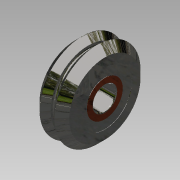
# Autodesk Inventor part: W3SSX
Saved by Autodesk Inventor 2020.1 (Build 241239000, 239)
## iProperties
Created: 2019-11-28
Part Number: W3SSX
Material: Generic
Catalog Web Link: https://www.bwc.com/dualvee.html
Description: Original DualVee Wheels-Original DualVee Wheels
Vendor: Bishop Wisecarver
Document SubType Name: Modeling
Designer: Autodesk Inc.
Manufacturer: BWC
Mass: 130.2 g
Surface Area: 59.8551 cm^2
Volume: 19.8505 cm^3
Density: 1 g/cm^3
Appearance: PSOLRGB-175-175-175
Category: FIRSTChoice
Company: Autodesk Inc.
PSOL_IDENT_0: {$CADENAS_DATA\23d-libs\bwc\dual_vee\wheels\original_dualvee_wheels.prj},168 {VTYP=3D},{NB=W3SSX},{L
PSOL_IDENT_1: INA=W3SSX},{NN=Original DualVee Wheels},{DATE=01.07.2019 05:07:11},{GEOMDATE=12.02.2019 13:07:27},{V
PSOL_IDENT_2: ERSION=},{LINEID=210},{WBVAR=},{WBNUMERIC=}  {NB=W3SSX},{LINA=W3SSX},{KT=DUMMY},{PN=W3SSX},{WS=WSSX
PSOL_IDENT_3: Stainless Steel Seal/Shield},{WSPN=SSX},{WSALG= 'X','WX Seal/Shield Steel', 'SSX','WSSX Seal/Shield
PSOL_IDENT_4: Stainless Steel','SS227', 'WSS227 Shield Stainless Steel Krytox GPL227 Lubricant','SS300', 'WSS300 S
PSOL_IDENT_5: tainless Steel Isoflex PDL 300 (grease, no shields or seals)','DW3SSX', 'Washdown Sealed Wheels' },{
PSOL_IDENT_6: SIZE=3},{D=1.803},{W=0.625},{B=0.4724},{VRI=0.750},{VRO=1.063},{WEIGHT=130.2},{C=0.755},{R=0.039},{R
PSOL_IDENT_7: 1=0.024},{E=0.010},{RLN=5900},{RLLBF=1326},{ALN=1701},{ALLBF=382},{ORMAT=440C Stainless steel},{IRMA
PSOL_IDENT_8: T=440C Stainless steel},{BMAT=440C Stainless steel},{RMAT=Nylon 6,6},{SHMAT=304 Stainless steel},{SM
PSOL_IDENT_9: AT=NBR+304 Stainless steel},{GREASE=Kluberplex BEM 34-132},{CFGFILTER=PN,WS,SIZE,D,W,B,VRI,VRO,WEIGH
PSOL_IDENT_10: T,RLN,RLLBF,ALN,ALLBF,ORMAT,IRMAT,BMAT,RMAT,SHMAT,SMAT,GREASE},{CATEGALG=Original Guide Wheel, Size
PSOL_IDENT_11: 3, Stainless Steel, Sealed/Shielded},{FEATALG=<li style=\" margin-top:0px; margin-bottom:0px; margin
PSOL_IDENT_12: -left:0px; margin-right:0px; -qt-block-indent:0; text-indent:0px;\"><span style=\" font-size:11pt; f
PSOL_IDENT_13: ont-weight:600;\">Corrosion resistant AISI 440C stainless steel</span></li><li style=\" font-size:11
PSOL_IDENT_14: pt; font-weight:600;\" style=\" margin-top:0px; margin-bottom:0px; margin-left:0px; margin-right:0px
PSOL_IDENT_15: ; -qt-block-indent:0; text-indent:0px;\">Double row angular contact ball bearing</li><li style=\" fo
PSOL_IDENT_16: nt-size:11pt; font-weight:600;\" style=\" margin-top:0px; margin-bottom:0px; margin-left:0px; margin
PSOL_IDENT_17: -right:0px; -qt-block-indent:0; text-indent:0px;\">Precision ground 90° vee inside or outside runnin
PSOL_IDENT_18: g surfaces</li><li style=\" font-size:11pt; font-weight:600;\" style=\" margin-top:0px; margin-botto
PSOL_IDENT_19: m:0px; margin-left:0px; margin-right:0px; -qt-block-indent:0; text-indent:0px;\">Hardened for heavy
PSOL_IDENT_20: loads and durability</li><li style=\" font-size:11pt; font-weight:600;\" style=\" margin-top:0px; ma
PSOL_IDENT_21: rgin-bottom:0px; margin-left:0px; margin-right:0px; -qt-block-indent:0; text-indent:0px;\">Seal/Shie
PSOL_IDENT_22: ld combination to protect against contamination</li>},{DESCRALG=<span style=\" font-size:11pt; font-
PSOL_IDENT_23: weight:600;\">DualVee WSSX series guide wheels are linear guide bearings with double row angular con
PSOL_IDENT_24: tact ball bearing arrangement.  Precision ground 90° vee inside or outside surfaces can be employed
PSOL_IDENT_25: to support loads and provide smooth and quiet motion. Use with DualVee guide track for linear motion
PSOL_IDENT_26: . Hybrid seal/shield design with rubber inner seal and metal outer shield protects against particle
PSOL_IDENT_27: contamination of all sizes. Through bore allows mounting on bushings or journals. Internally lubrica
PSOL_IDENT_28: ted with general purpose grease. </span>},{RATINGSALG=<span style=\" font-size:11pt; font-weight:600
PSOL_IDENT_29: ; color:#000000;\">Temperature Range:</span><span style=\" font-size:11pt; color:#000000;\"> -22°F t
PSOL_IDENT_30: o +212°F</span></p><p style=\" margin-top:0px; margin-bottom:0px; margin-left:0px; margin-right:0px;
PSOL_IDENT_31: -qt-block-indent:0; text-indent:0px;\"><span style=\" font-size:11pt; font-weight:600; color:#00000
PSOL_IDENT_32: 0;\">RoHS Compliant</span>},{MATCOLALG=ORMAT( title=\"$var. ($desc.)\", format=\"$value(SRC=VALDESC)
PSOL_IDENT_33: .\" ),IRMAT( title=\"$var. ($desc.)\", format=\"$value(SRC=VALDESC).\" ),BMAT( title=\"$var. ($desc.
PSOL_IDENT_34: )\", format=\"$value(SRC=VALDESC).\" ),RMAT( title=\"$var. ($desc.)\", format=\"$value(SRC=VALDESC).
PSOL_IDENT_35: \" ),SHMAT( title=\"$var. ($desc.)\", format=\"$value(SRC=VALDESC).\" ),SMAT( title=\"$var. ($desc.)
PSOL_IDENT_36: \", format=\"$value(SRC=VALDESC).\" ),GREASE( title=\"$var. ($desc.)\", format=\"$value(SRC=VALDESC)
PSOL_IDENT_37: .\" )},{MATCOL1=ORMAT( title=\"$var. ($desc.)\", format=\"$value(SRC=VALDESC).\" ),IRMAT( title=\"$v
PSOL_IDENT_38: ar. ($desc.)\", format=\"$value(SRC=VALDESC).\" ),BMAT( title=\"$var. ($desc.)\", format=\"$value(SR
PSOL_IDENT_39: C=VALDESC).\" ),RMAT( title=\"$var. ($desc.)\", format=\"$value(SRC=VALDESC).\" ),SHMAT( title=\"$va
PSOL_IDENT_40: r. ($desc.)\", format=\"$value(SRC=VALDESC).\" ),SMAT( title=\"$var. ($desc.)\", format=\"$value(SRC=
PSOL_IDENT_41: VALDESC).\" ),GREASE( title=\"$var. ($desc.)\", format=\"$value(SRC=VALDESC).\" )}
NN: Original DualVee Wheels
NT: Original DualVee Wheels
NB: W3SSX
NBSYN: $PN.
LINA: W3SSX
PN: W3SSX
WS: WSSX Stainless Steel Seal/Shield
SIZE: 3
D: 1.803
W: 0.625
B: 0.4724
VRI: 0.75
VRO: 1.063
WEIGHT: 130.2
RLN: 5900
RLLBF: 1326
ALN: 1701
ALLBF: 382
ORMAT: 440C Stainless steel
IRMAT: 440C Stainless steel
BMAT: 440C Stainless steel
RMAT: Nylon 6,6
SHMAT: 304 Stainless steel
SMAT: NBR+304 Stainless steel
GREASE: Kluberplex BEM 34-132
SUPPLIER: BWC
ARTICLENO: W3SSX
BOMINFO: W3SSX
CREATOR: CADENAS GmbH
Title: W3SSX
Author: Autodesk Inc.
Comments: Original DualVee Wheels
Autodesk Inventor part; units mm, degrees
sketch "Sketch_1" plane through (0, 0, 0) normal (0, 0, 1) x (1, 0, 0)
  line L0 (7.3279, 0) -> (-7.3279, 0)
  line L1 (-7.9375, 9.5885) -> (-7.9375, 6.6091)
  arc A0 (-7.9375, 6.6091) -> (-7.3279, 5.9995) centre (-7.3279, 6.6091) ccw
  line L2 (-7.3279, 5.9995) -> (7.3279, 5.9995)
  arc A1 (7.3279, 5.9995) -> (7.9375, 6.6091) centre (7.3279, 6.6091) ccw
  line L3 (7.9375, 6.6091) -> (7.9375, 9.5885)
  line L4 (7.9375, 9.5885) -> (7.8105, 9.5885)
  line L5 (7.8105, 9.5885) -> (7.8105, 9.4615)
  line L6 (7.8105, 9.4615) -> (7.6835, 9.4615)
  line L7 (7.6835, 9.4615) -> (7.6835, 14.4463)
  line L8 (7.6835, 14.4463) -> (7.8105, 14.4463)
  line L9 (7.8105, 14.4463) -> (7.8105, 14.3193)
  line L10 (7.8105, 14.3193) -> (7.9375, 14.3193)
  line L11 (7.9375, 14.3193) -> (7.9375, 19.05)
  line L12 (7.9375, 19.05) -> (4.0894, 22.8981)
  line L13 (4.0894, 22.8981) -> (3.8354, 22.8981)
  line L14 (3.8354, 22.8981) -> (0.9906, 20.0533)
  line L15 (0.9906, 20.0533) -> (0.9906, 19.05)
  arc A2 (-0.9906, 19.05) -> (0.9906, 19.05) centre (0, 19.05) ccw
  line L16 (-0.9906, 19.05) -> (-0.9906, 20.0533)
  line L17 (-0.9906, 20.0533) -> (-3.8354, 22.8981)
  line L18 (-3.8354, 22.8981) -> (-4.0894, 22.8981)
  line L19 (-4.0894, 22.8981) -> (-7.9375, 19.05)
  line L20 (-7.9375, 19.05) -> (-7.9375, 14.3193)
  line L21 (-7.9375, 14.3193) -> (-7.8105, 14.3193)
  line L22 (-7.8105, 14.3193) -> (-7.8105, 14.4463)
  line L23 (-7.8105, 14.4463) -> (-7.6835, 14.4463)
  line L24 (-7.6835, 14.4463) -> (-7.6835, 9.4615)
  line L25 (-7.6835, 9.4615) -> (-7.8105, 9.4615)
  line L26 (-7.8105, 9.4615) -> (-7.8105, 9.5885)
  line L27 (-7.8105, 9.5885) -> (-7.9375, 9.5885)
  constraints: 56 end point, 6 point on circle, 3 centre point
revolve "Revolution1" add sketch "Sketch_1" angle 360 about axis through (7.3279, 0, 0) along (1, 0, 0)
ref_plane "b_XY" through (-7.3279, 5.9995, 0) normal (0, 0, 1) x (1, 0, 0)
ref_plane "b_YZ" through (-7.3279, 5.9995, 0) normal (1, 0, 0) x (0, 1, 0)
ref_plane "b_ZX" through (-7.3279, 5.9995, 0) normal (0, 1, 0) x (0, 0, 1)
ref_plane "b1_XY" through (-7.3279, -5.9995, 0) normal (0, 0, 1) x (1, 0, 0)
ref_plane "b1_YZ" through (-7.3279, -5.9995, 0) normal (1, 0, 0) x (0, 1, 0)
ref_plane "b1_ZX" through (-7.3279, -5.9995, 0) normal (0, 1, 0) x (0, 0, 1)
ref_plane "d_XY" through (-3.9688, 22.8981, 0) normal (0, 0, 1) x (1, 0, 0)
ref_plane "d_YZ" through (-3.9688, 22.8981, 0) normal (1, 0, 0) x (0, 1, 0)
ref_plane "d_ZX" through (-3.9688, 22.8981, 0) normal (0, 1, 0) x (0, 0, 1)
ref_plane "d1_XY" through (-3.9688, -22.8981, 0) normal (0, 0, 1) x (1, 0, 0)
ref_plane "d1_YZ" through (-3.9688, -22.8981, 0) normal (1, 0, 0) x (0, 1, 0)
ref_plane "d1_ZX" through (-3.9688, -22.8981, 0) normal (0, 1, 0) x (0, 0, 1)
ref_plane "vri_XY" through (0, 19.05, 0) normal (0, 0, 1) x (1, 0, 0)
ref_plane "vri_YZ" through (0, 19.05, 0) normal (1, 0, 0) x (0, 1, 0)
ref_plane "vri_ZX" through (0, 19.05, 0) normal (0, 1, 0) x (0, 0, 1)
ref_plane "vri1_XY" through (7.9375, 0, 0) normal (0, 0, 1) x (1, 0, 0)
ref_plane "vri1_YZ" through (7.9375, 0, 0) normal (1, 0, 0) x (0, 1, 0)
ref_plane "vri1_ZX" through (7.9375, 0, 0) normal (0, 1, 0) x (0, 0, 1)
ref_plane "w_XY" through (-7.9375, 19.05, 0) normal (0, 0, 1) x (1, 0, 0)
ref_plane "w_YZ" through (-7.9375, 19.05, 0) normal (1, 0, 0) x (0, 1, 0)
ref_plane "w_ZX" through (-7.9375, 19.05, 0) normal (0, 1, 0) x (0, 0, 1)
ref_plane "w1_XY" through (7.9375, 19.05, 0) normal (0, 0, 1) x (1, 0, 0)
ref_plane "w1_YZ" through (7.9375, 19.05, 0) normal (1, 0, 0) x (0, 1, 0)
ref_plane "w1_ZX" through (7.9375, 19.05, 0) normal (0, 1, 0) x (0, 0, 1)
ref_plane "wheel_XY" through (7.9375, 0, 0) normal (1, 0, 0) x (0, 0, -1)
ref_plane "wheel_YZ" through (7.9375, 0, 0) normal (0, 0, -1) x (0, 1, 0)
ref_plane "wheel_ZX" through (7.9375, 0, 0) normal (0, 1, 0) x (1, 0, 0)
ref_plane "wheel2_XY" through (-7.9375, 0, 0) normal (1, 0, 0) x (0, 0, -1)
ref_plane "wheel2_YZ" through (-7.9375, 0, 0) normal (0, 0, -1) x (0, 1, 0)
ref_plane "wheel2_ZX" through (-7.9375, 0, 0) normal (0, 1, 0) x (1, 0, 0)
body "Solid1"
